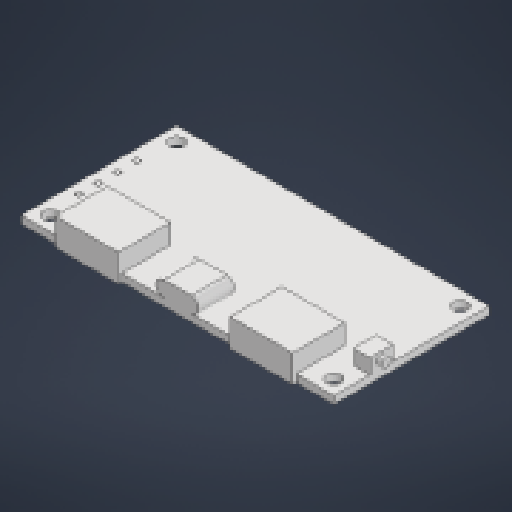
# Autodesk Inventor part: circuit board
Saved by Autodesk Inventor 2026.2 (Build 302298010, 298A)
## iProperties
Created: 2026-03-13
Part Number: circuit board
Material: 一般
Document SubType Name: Modeling
Designer: gavin
Density: 1 g/cm^3
Appearance: 預設
Author: gavin
Autodesk Inventor part; units mm, degrees
ref_plane "YZ Plane" through (0, 0, 0) normal (1, 0, 0) x (0, 1, 0)
ref_plane "XZ Plane" through (0, 0, 0) normal (0, 1, 0) x (-1, 0, 0)
ref_plane "XY Plane" through (0, 0, 0) normal (0, 0, 1) x (1, 0, 0)
sketch "草圖1" plane through (0, 0, 0) normal (0, 1, 0) x (-1, 0, 0)
  line L0 (0, 0) -> (-65, 0)
  line L1 (-65, 0) -> (-65, -32.3)
  line L2 (-65, -32.3) -> (0, -32.3)
  line L3 (0, -32.3) -> (0, 0)
  circle A0 centre (-3, -3) radius 1.5
  circle A1 centre (-3, -29.3) radius 1.5
  circle A2 centre (-62, -3) radius 1.5
  circle A3 centre (-62, -29.3) radius 1.5
  dimension "d0" = 65
  dimension "d1" = 32.3
  dimension "d4" = 3
  dimension "d5" = 3
  dimension "d6" = 3
  dimension "d7" = 3
  dimension "d8" = 3
  dimension "d9" = 3
  dimension "d10" = 3
  dimension "d11" = 3
  dimension "d12" = 3
  dimension "d13" = 3
  dimension "d14" = 3
  dimension "d15" = 3
  constraints: 8 end point, 4 centre point, 2 parallel, 1 horizontal, 1 perpendicular
  measures "d0" distance of L2.end L1.end
  measures "d1" distance of L1.end L0.end
  measures "d4" diameter of A0
  measures "d5" distance from line of L3 A0.centre
  measures "d6" distance from line of L0 A0.centre
  measures "d7" diameter of A1
  measures "d8" diameter of A2
  measures "d9" diameter of A3
  measures "d10" distance from line of L1 A2.centre
  measures "d11" distance from line of L0 A2.centre
  measures "d12" distance from line of L2 A3.centre
  measures "d13" distance from line of L1 A3.centre
  measures "d14" distance from line of L3 A1.centre
  measures "d15" distance from line of L2 A1.centre
extrude "擠出1" add sketch "草圖1" along normal blind 1.6
sketch "草圖2" plane through (0, 0, 0) normal (0, 0, 1) x (1, 0, 0)
  line L0 (0, 0) -> (65, 0) projected
  line L1 (65, 0) -> (65, 1.6) projected
  line L2 (0, 1.6) -> (65, 1.6) projected
  line L3 (0, 0) -> (0, 1.6) projected
  line L4 (7.88, 0) -> (20.91, 0)
  line L5 (20.91, 0) -> (20.91, 5.7)
  line L6 (20.91, 5.7) -> (7.88, 5.7)
  line L7 (7.88, 5.7) -> (7.88, 0)
  line L8 (44.09, 0) -> (57.12, 0)
  line L9 (57.12, 0) -> (57.12, 5.7)
  line L10 (57.12, 5.7) -> (44.09, 5.7)
  line L11 (44.09, 5.7) -> (44.09, 0)
  point P0 (44.09, 1.6)
  point P1 (57.12, 1.6)
  dimension "d16" = 13.03
  dimension "d17" = 5.7
  dimension "d18" = 13.03
  dimension "d19" = 5.7
  dimension "d20" = 7.88
  dimension "d21" = 7.88
  constraints: 16 end point, 4 parallel, 2 horizontal, 2 perpendicular, 2 point on line
  measures "d16" distance of L5.end L6.end
  measures "d17" distance between parallel lines of L0 L6
  measures "d18" distance of L9.end L10.end
  measures "d19" distance of L10.end L8.start
  measures "d20" distance between parallel lines of L3 L7
  measures "d21" distance between parallel lines of L1 L9
extrude "擠出2" add sketch "草圖2" along normal blind 0.7 contours L7 L2 L5 L0 | L7 L6 L5 L2 | L11 L2 L9 L0 | L11 L10 L9 L2
sketch "草圖3" plane through (0, 0, 0) normal (0, 0, -1) x (-1, 0, 0)
  line L0 (-7.88, 1.6) -> (-20.91, 1.6) projected
  line L1 (-7.88, 5.7) -> (-7.88, 1.6) projected
  line L2 (-20.91, 5.7) -> (-7.88, 5.7) projected
  line L3 (-20.91, 1.6) -> (-20.91, 5.7) projected
  line L4 (-57.12, 5.7) -> (-44.09, 5.7) projected
  line L5 (-44.09, 5.7) -> (-44.09, 1.6) projected
  line L6 (-57.12, 5.7) -> (-44.09, 5.7) projected
  line L7 (-57.12, 1.6) -> (-57.12, 5.7) projected
  line L8 (-7.88, 1.6) -> (-20.91, 1.6) projected
  line L9 (-7.88, 5.7) -> (-7.88, 1.6) projected
  line L10 (-20.91, 5.7) -> (-7.88, 5.7) projected
  line L11 (-20.91, 1.6) -> (-20.91, 5.7) projected
  line L12 (-44.09, 1.6) -> (-57.12, 1.6) projected
  point P0 (0, 0)
extrude "擠出3" add sketch "草圖3" along normal blind 10.1
sketch "草圖4" plane through (65, 0, 0) normal (0, 0, 1) x (1, 0, 0)
  line L0 (-44.09, 1.6) -> (-44.09, 0) projected
  line L1 (-65, 0) -> (-57.12, 0) projected
  line L2 (0, 0) -> (0, 1.6) projected
  line L3 (-7.88, 1.6) -> (0, 1.6) projected
  line L4 (-65, 1.6) -> (-57.12, 1.6) projected
  line L5 (-44.09, 1.6) -> (-20.91, 1.6) projected
  line L6 (-35.37, 1.6) -> (-29.63, 1.6)
  line L7 (-28.03, 3.2) -> (-28.03, 3.2)
  line L8 (-29.63, 4.8) -> (-35.37, 4.8)
  line L9 (-36.97, 3.2) -> (-36.97, 3.2)
  arc A0 (-35.37, 4.8) -> (-36.97, 3.2) centre (-35.37, 3.2) ccw
  arc A1 (-36.97, 3.2) -> (-35.37, 1.6) centre (-35.37, 3.2) ccw
  arc A2 (-29.63, 1.6) -> (-28.03, 3.2) centre (-29.63, 3.2) ccw
  arc A3 (-28.03, 3.2) -> (-29.63, 4.8) centre (-29.63, 3.2) ccw
  line L10 (0, 0) -> (-65, 0) projected
  line L11 (-57.12, 0) -> (-57.12, 1.6) projected
  line L12 (-65, 0) -> (-65, 1.6) projected
  line L13 (-44.09, 0) -> (-20.91, 0) projected
  line L14 (-20.91, 0) -> (-20.91, 1.6) projected
  line L15 (-7.88, 1.6) -> (-7.88, 0) projected
  line L16 (-7.88, 0) -> (0, 0) projected
  point P0 (-36.97, 1.6)
  point P1 (-28.03, 4.8)
  point P2 (-28.03, 1.6)
  point P3 (-36.97, 4.8)
  point P4 (-32.5, 4.8)
  point P5 (-32.5, 0)
  point P6 (-35.37, 1.6)
  point P7 (-29.63, 1.6)
  dimension "d26" = 8.94
  dimension "d27" = 3.2
  dimension "d28" = 1.6
  constraints: 9 point on line, 8 end point, 8 point on circle, 8 tangent, 4 centre point, 3 equal radius, 2 midpoint, 2 parallel, 1 horizontal, 1 perpendicular, 1 vertical alignment
  measures "d26" distance of point (-28.03, 4.8) point (-36.97, 4.8)
  measures "d27" distance of point (-28.03, 1.6) point (-28.03, 4.8)
  measures "d28" radius of A0
extrude "擠出4" add sketch "草圖4" against normal blind 7.4 contours A1 A0 L8 A3 A2 L5
sketch "草圖5" plane through (65, 0, 0) normal (1, 0, 0) x (0, 0, -1)
  line L0 (0, 0) -> (32.3, 0) projected
  line L1 (32.3, 0) -> (32.3, 1.6) projected
  line L2 (0, 1.6) -> (32.3, 1.6) projected
  line L3 (0, 0) -> (0, 1.6) projected
  line L4 (7.5, 1.6) -> (12.2, 1.6)
  line L5 (12.2, 1.6) -> (12.2, 4.7)
  line L6 (12.2, 4.7) -> (7.5, 4.7)
  line L7 (7.5, 4.7) -> (7.5, 1.6)
  dimension "d31" = 4.7
  dimension "d32" = 3.1
  dimension "d33" = 7.5
  constraints: 8 end point, 2 parallel, 1 horizontal, 1 perpendicular, 1 point on line
  measures "d31" distance of L6.end L5.end
  measures "d32" distance of L5.end L4.end
  measures "d33" distance between parallel lines of L3 L7
extrude "擠出5" add sketch "草圖5" against normal blind 3.4 contours L7 L6 L5 L2
sketch "草圖6" plane through (65, 0, 0) normal (1, 0, 0) x (0, 0, -1)
  line L0 (0, 0) -> (32.3, 0) projected
  line L1 (32.3, 0) -> (32.3, 1.6) projected
  line L2 (12.2, 1.6) -> (32.3, 1.6) projected
  line L3 (12.2, 1.6) -> (12.2, 4.7) projected
  line L4 (12.2, 4.7) -> (7.5, 4.7) projected
  line L5 (7.5, 4.7) -> (7.5, 1.6) projected
  line L6 (0, 1.6) -> (7.5, 1.6) projected
  line L7 (0, 0) -> (0, 1.6) projected
  line L8 (7.5, 1.6) -> (12.2, 1.6)
  circle A0 centre (9.85, 3.19) radius 0.95
  dimension "d36" = 1.9
  constraints: 2 end point, 1 centre point, 1 horizontal
  measures "d36" diameter of A0
extrude "擠出6" add sketch "草圖6" along normal blind 1 contours A0
sketch "草圖7" plane through (0, 1.6, 0) normal (0, 1, 0) x (1, 0, 0)
  circle A0 centre (62, 29.3) radius 1.5 projected
  circle A1 centre (62, 3) radius 1.5 projected
  circle A2 centre (3, 29.3) radius 1.5 projected
  circle A3 centre (3, 3) radius 1.5 projected
  line L0 (65, 7.5) -> (61.6, 7.5) projected
  line L1 (61.6, 7.5) -> (61.6, 12.2) projected
  line L2 (61.6, 12.2) -> (65, 12.2) projected
  line L3 (65, 12.2) -> (65, 32.3) projected
  line L4 (65, 32.3) -> (0, 32.3) projected
  line L5 (0, 32.3) -> (0, 0) projected
  line L6 (0, 0) -> (7.88, 0) projected
  line L7 (7.88, 0) -> (7.88, 10.1) projected
  line L8 (7.88, 10.1) -> (20.91, 10.1) projected
  line L9 (20.91, 10.1) -> (20.91, 0) projected
  line L10 (20.91, 0) -> (29.63, 0) projected
  line L11 (29.63, 0) -> (29.63, 7.4) projected
  line L12 (29.63, 7.4) -> (35.37, 7.4) projected
  line L13 (35.37, 0) -> (35.37, 7.4) projected
  line L14 (35.37, 0) -> (44.09, 0) projected
  line L15 (44.09, 0) -> (44.09, 10.1) projected
  line L16 (44.09, 10.1) -> (57.12, 10.1) projected
  line L17 (57.12, 10.1) -> (57.12, 0) projected
  line L18 (57.12, 0) -> (65, 0) projected
  line L19 (65, 0) -> (65, 7.5) projected
  line L20 (1.8, 22.24) -> (2.8, 22.24)
  line L21 (2.8, 22.24) -> (2.8, 21.24)
  line L22 (2.8, 21.24) -> (1.8, 21.24)
  line L23 (1.8, 21.24) -> (1.8, 22.24)
  line L24 (1.8, 22.24) -> (2.8, 21.24) construction
  line L25 (2.8, 22.24) -> (1.8, 21.24) construction
  line L26 (1.8, 10.24) -> (2.8, 10.24)
  line L27 (2.8, 10.24) -> (2.8, 9.24)
  line L28 (2.8, 9.24) -> (1.8, 9.24)
  line L29 (1.8, 9.24) -> (1.8, 10.24)
  line L30 (1.8, 10.24) -> (2.8, 9.24) construction
  line L31 (2.8, 10.24) -> (1.8, 9.24) construction
  line L32 (1.8, 14.24) -> (2.8, 14.24)
  line L33 (2.8, 14.24) -> (2.8, 13.24)
  line L34 (2.8, 13.24) -> (1.8, 13.24)
  line L35 (1.8, 13.24) -> (1.8, 14.24)
  line L36 (1.8, 14.24) -> (2.8, 13.24) construction
  line L37 (2.8, 14.24) -> (1.8, 13.24) construction
  line L38 (1.8, 17.24) -> (2.8, 17.24)
  line L39 (2.8, 17.24) -> (2.8, 18.24)
  line L40 (2.8, 18.24) -> (1.8, 18.24)
  line L41 (1.8, 18.24) -> (1.8, 17.24)
  line L42 (1.8, 17.24) -> (2.8, 18.24) construction
  line L43 (2.8, 17.24) -> (1.8, 18.24) construction
  point P0 (2.3, 21.74)
  point P1 (2.3, 9.74)
  point P2 (2.3, 13.74)
  point P3 (2.3, 17.74)
  point P4 (2.3, 17.24)
  dimension "d39" = 1
  dimension "d40" = 1
  dimension "d41" = 1
  dimension "d42" = 1
  dimension "d43" = 1
  dimension "d44" = 1
  dimension "d45" = 1
  dimension "d46" = 1
  dimension "d47" = 2.3
  dimension "d48" = 10.56
  dimension "d55" = 4
  dimension "d56" = 4
  dimension "d57" = 4
  constraints: 48 end point, 9 midpoint, 8 parallel, 4 horizontal, 4 perpendicular, 3 vertical alignment
  measures "d39" distance of L21.end L22.end
  measures "d40" distance of L20.end L21.end
  measures "d41" distance of L27.end L28.end
  measures "d42" distance of L26.end L27.end
  measures "d43" distance of L33.end L34.end
  measures "d44" distance of L32.end L33.end
  measures "d45" distance of L40.end L39.end
  measures "d46" distance of L39.end L38.end
  measures "d47" distance from line of L5 point (2.3, 21.74)
  measures "d48" distance from line of L4 point (2.3, 21.74)
  measures "d55" distance of point (2.3, 17.74) point (2.3, 21.74)
  measures "d56" distance of point (2.3, 13.74) point (2.3, 17.74)
  measures "d57" distance of point (2.3, 9.74) point (2.3, 13.74)
extrude "擠出7" add sketch "草圖7" along normal blind 0.1 contours L20 L21 L22 L23 | L26 L27 L28 L29 | L32 L33 L34 L35 | L41 L40 L39 L38
equation "\"d18\" = d16"
equation "\"d19\" = d17"
equation "\"d21\" = d20"
